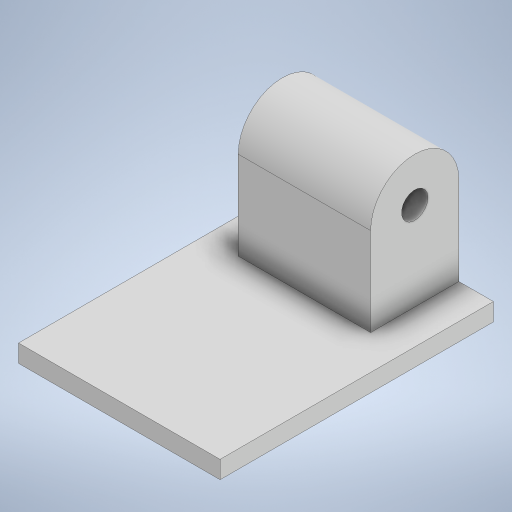
# Autodesk Inventor part: uchwyt
Saved by Autodesk Inventor 2023 (Build 270158000, 158)
## iProperties
Created: 2024-05-12
Part Number: uchwyt
Material: Ogólny
Document SubType Name: Modeling
Designer: kamil
Density: 1 g/cm^3
Appearance: Domyślna
Author: kamil
Autodesk Inventor part; units mm, degrees
ref_plane "YZ Plane" through (0, 0, 0) normal (1, 0, 0) x (0, 1, 0)
ref_plane "XZ Plane" through (0, 0, 0) normal (0, 1, 0) x (-1, 0, 0)
ref_plane "XY Plane" through (0, 0, 0) normal (0, 0, 1) x (1, 0, 0)
sketch "Szkic1" plane through (0, 0, 0) normal (0, 1, 0) x (-1, 0, 0)
  line L0 (11.7026, 13.5166) -> (-11.1274, 13.5166)
  line L1 (-11.1274, 13.5166) -> (-11.1274, -17.4543)
  line L2 (-11.1274, -17.4543) -> (11.7026, -17.4543)
  line L3 (11.7026, -17.4543) -> (11.7026, 13.5166)
  point P0 (0, 0)
  constraints: 8 end point, 2 parallel, 1 horizontal, 1 perpendicular
extrude "Wyciągnięcie proste1" add sketch "Szkic1" along normal blind 2
sketch "Szkic2" plane through (0, 2, 0) normal (0, 1, 0) x (1, 0, 0)
  line L0 (11.1274, 17.4543) -> (-11.7026, 17.4543) projected
  line L1 (-7.7876, 7.4543) -> (7.2124, 7.4543)
  line L2 (7.2124, 7.4543) -> (7.2124, 17.4543)
  line L3 (7.2124, 17.4543) -> (-7.7876, 17.4543)
  line L4 (-7.7876, 17.4543) -> (-7.7876, 7.4543)
  point P0 (0, 0)
  point P1 (-0.2876, 7.4543)
  point P2 (-0.2876, 17.4543)
  dimension "d2" = 15
  dimension "d3" = 10
  constraints: 8 end point, 2 midpoint, 2 parallel, 1 horizontal, 1 perpendicular, 1 point on line, 1 vertical alignment
  measures "d2" distance of L1.start L1.end
  measures "d3" distance of L3.end L1.start
extrude "Wyciągnięcie proste2" add sketch "Szkic2" along normal blind 15
fillet "Zaokrąglenie1" radius 5 2 edges at (-0.2876, 17, -7.4543) (-0.2876, 17, -17.4543)
sketch "Szkic3" plane through (7.2124, 2, -7.4543) normal (1, 0, 0) x (0, 0, -1)
  arc A0 (10, 10) -> (0, 10) centre (5, 10) ccw projected
  line L0 (0, 0) -> (0, 10) projected
  line L1 (10, 0) -> (0, 0) projected
  line L2 (10, 0) -> (10, 10) projected
  circle A1 centre (5, 10) radius 1.5
  point P0 (-7.4543, -2)
  dimension "d7" = 3
  constraints: 1 centre point, 1 coincident
  measures "d7" diameter of A1
extrude "Wyciągnięcie proste3" cut sketch "Szkic3" against normal blind 15 contours A1
